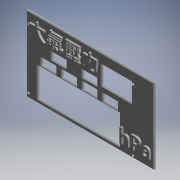
# Autodesk Inventor part: 大氣壓力
Saved by Autodesk Inventor 2021 (Build 250183000, 183)
## iProperties
Part Number: 大氣壓力
Material: 一般
Document SubType Name: 塑型
Designer: aura0
Appearance: 預設
Author: aura0
Autodesk Inventor part; units mm, degrees
ref_plane "YZ 平面" through (0, 0, 0) normal (1, 0, 0) x (0, 1, 0)
ref_plane "XZ 平面" through (0, 0, 0) normal (0, 1, 0) x (-1, 0, 0)
ref_plane "XY 平面" through (0, 0, 0) normal (0, 0, 1) x (1, 0, 0)
sketch "草圖1" plane through (0, 0, 0) normal (0, 0, 1) x (1, 0, 0)
  line L0 (-95, 56.05) -> (95, 56.05)
  line L1 (95, 56.05) -> (95, -56.05)
  line L2 (95, -56.05) -> (-95, -56.05)
  line L3 (-95, -56.05) -> (-95, 56.05)
  line L4 (-95, 56.05) -> (95, -56.05) construction
  line L5 (95, 56.05) -> (-95, -56.05) construction
  point P0 (0, 0)
  dimension "d0" = 190
  dimension "d1" = 112.1
  constraints: 12 end point, 2 midpoint, 2 parallel, 1 horizontal, 1 perpendicular
  measures "d0" distance of L1.end L2.end
  measures "d1" distance of L0.end L1.end
extrude "擠出1" add sketch "草圖1" along normal blind 3
sketch "草圖2" plane through (0, 0, 3) normal (0, 0, 1) x (1, 0, 0)
  line L0 (-78.4, -50.75) -> (43.6, -50.75)
  line L1 (43.6, -50.75) -> (43.6, -7.75)
  line L2 (43.6, -7.75) -> (-78.4, -7.75)
  line L3 (-78.4, -7.75) -> (-78.4, -50.75)
  line L4 (-95, 56.05) -> (-95, -56.05) projected
  line L5 (-95, -56.05) -> (95, -56.05) projected
  line L6 (17.1, 13.68) -> (61.5, 13.68)
  line L7 (61.5, 13.68) -> (61.5, 41.38)
  line L8 (61.5, 41.38) -> (17.1, 41.38)
  line L9 (17.1, 41.38) -> (17.1, 13.68)
  line L10 (-72.8, -5.05) -> (-51.2, -5.05)
  line L11 (-51.2, -5.05) -> (-51.2, 5.15)
  line L12 (-51.2, 5.15) -> (-72.8, 5.15)
  line L13 (-72.8, 5.15) -> (-72.8, -5.05)
  line L14 (-42.2, -5.05) -> (-20.6, -5.05)
  line L15 (-20.6, -5.05) -> (-20.6, 5.15)
  line L16 (-20.6, 5.15) -> (-42.2, 5.15)
  line L17 (-42.2, 5.15) -> (-42.2, -5.05)
  line L18 (-11.6, -5.05) -> (10, -5.05)
  line L19 (10, -5.05) -> (10, 5.15)
  line L20 (10, 5.15) -> (-11.6, 5.15)
  line L21 (-11.6, 5.15) -> (-11.6, -5.05)
  line L22 (19, -5.05) -> (40.6, -5.05)
  line L23 (40.6, -5.05) -> (40.6, 5.15)
  line L24 (40.6, 5.15) -> (19, 5.15)
  line L25 (19, 5.15) -> (19, -5.05)
  line L26 (-57.5, 20.25) -> (-35.9, 20.25)
  line L27 (-35.9, 20.25) -> (-35.9, 10.05)
  line L28 (-35.9, 10.05) -> (-57.5, 10.05)
  line L29 (-57.5, 10.05) -> (-57.5, 20.25)
  line L30 (-11.8, 20.25) -> (9.8, 20.25)
  line L31 (9.8, 20.25) -> (9.8, 10.05)
  line L32 (9.8, 10.05) -> (-11.8, 10.05)
  line L33 (-11.8, 10.05) -> (-11.8, 20.25)
  point P0 (0, 0)
  dimension "d54" = 159
  dimension "d4" = 16.6
  dimension "d5" = 5.3
  dimension "d6" = 122
  dimension "d7" = 43
  dimension "d8" = 51
  dimension "d9" = 22.2
  dimension "d10" = 21.6
  dimension "d11" = 10.2
  dimension "d12" = 21.6
  dimension "d13" = 21.6
  dimension "d14" = 21.6
  dimension "d17" = 10.2
  dimension "d18" = 10.2
  dimension "d19" = 10.2
  dimension "d22" = 9
  dimension "d23" = 9
  dimension "d25" = 9
  dimension "d29" = 37.5
  dimension "d30" = 66.1
  dimension "d31" = 24.1
  dimension "d32" = 10.2
  dimension "d33" = 10.2
  dimension "d34" = 21.6
  dimension "d35" = 21.6
  dimension "d36" = 4.9
  dimension "d37" = 4.9
  dimension "d38" = 69.73
  dimension "d39" = 112.1
  dimension "d40" = 44.4
  dimension "d41" = 27.7
  constraints: 64 end point, 16 parallel, 8 horizontal, 8 perpendicular, 5 point on line
  measures "d4" distance between parallel lines of L4 L3
  measures "d5" distance between parallel lines of L5 L0
  measures "d6" distance of L0.start L0.end
  measures "d7" distance of L2.end L0.start
  measures "d8" distance between parallel lines of L5 L10
  measures "d9" distance between parallel lines of L4 L13
  measures "d10" distance of L10.start L10.end
  measures "d11" distance of L12.end L10.start
  measures "d12" distance of L14.start L14.end
  measures "d13" distance of L18.start L18.end
  measures "d14" distance of L22.start L22.end
  measures "d17" distance of L14.end L15.end
  measures "d18" distance of L18.end L19.end
  measures "d19" distance of L22.end L23.end
  measures "d22" distance between parallel lines of L17 L11
  measures "d23" distance between parallel lines of L21 L15
  measures "d25" distance between parallel lines of L25 L19
  measures "d29" distance between parallel lines of L4 L29
  measures "d30" distance between parallel lines of L5 L28
  measures "d31" distance between parallel lines of L27 L33
  measures "d32" distance of L28.end L26.start
  measures "d33" distance of L32.end L30.start
  measures "d34" distance of L27.end L28.end
  measures "d35" distance of L31.end L32.end
  measures "d36" distance between parallel lines of L16 L28
  measures "d37" distance between parallel lines of L20 L32
  measures "d38" distance between parallel lines of L5 L6
  measures "d39" distance between parallel lines of L4 L9
  measures "d40" distance of L6.start L6.end
  measures "d41" distance of L6.end L7.end
extrude "擠出2" cut sketch "草圖2" against normal blind 3
sketch "草圖3" plane through (0, 0, 3) normal (0, 0, 1) x (1, 0, 0)
  line L0 (-90.6336, 50.0448) -> (-11.3203, 50.0448) construction
  line L1 (-11.3203, 50.0448) -> (-11.3203, 32.4568) construction
  line L2 (-11.3203, 32.4568) -> (-90.6336, 32.4568) construction
  line L3 (-90.6336, 32.4568) -> (-90.6336, 50.0448) construction
  line L4 (44.7132, -22.7639) -> (92.593, -22.7639) construction
  line L5 (92.593, -22.7639) -> (92.593, -44.2402) construction
  line L6 (92.593, -44.2402) -> (44.7132, -44.2402) construction
  line L7 (44.7132, -44.2402) -> (44.7132, -22.7639) construction
  line L8 (-65.6723, 28.4482) -> (-67.0972, 26.5426)
  spline S0 degree 2 poles (-67.0972, 26.5426) (-74.9427, 31.5383) (-77.2774, 39.8302) knots 0 0 0 1 1 1
  spline S1 degree 2 poles (-77.2774, 39.8302) (-79.7495, 31.8474) (-87.595, 26.7315) knots 0 0 0 1 1 1
  line L9 (-87.595, 26.7315) -> (-88.9856, 28.7744)
  spline S2 degree 2 poles (-88.9856, 28.7744) (-80.8997, 34.062) (-79.1315, 41.7186) knots 0 0 0 1 1 1
  line L10 (-79.1315, 41.7186) -> (-88.4362, 41.7186)
  line L11 (-88.4362, 41.7186) -> (-88.4706, 44.0877)
  line L12 (-88.4706, 44.0877) -> (-78.8225, 44.0877)
  spline S3 degree 2 poles (-78.8225, 44.0877) (-78.5306, 46.8688) (-78.4963, 49.7529) knots 0 0 0 1 1 1
  line L13 (-78.4963, 49.7529) -> (-76.1272, 49.7529)
  spline S4 degree 2 poles (-76.1272, 49.7529) (-76.1615, 46.3023) (-76.3504, 44.0877) knots 0 0 0 1 1 1
  line L14 (-76.3504, 44.0877) -> (-66.0156, 44.0877)
  line L15 (-66.0156, 44.0877) -> (-66.0156, 41.7186)
  line L16 (-66.0156, 41.7186) -> (-75.595, 41.7186)
  spline S5 degree 2 poles (-75.595, 41.7186) (-73.6551, 33.2036) (-65.6723, 28.4482) knots 0 0 0 1 1 1
  spline S6 degree 2 poles (-39.0972, 31.9332) (-39.4233, 29.4783) (-40.7967, 26.6456) (-42.05, 26.6456) knots 0 0 0 1 2 2 2
  spline S7 degree 2 poles (-42.05, 26.6456) (-42.8912, 26.6456) (-44.1615, 27.9847) (-45.1229, 33.3238) (-45.1229, 37.3066) knots 0 0 0 1 2 3 3 3
  spline S8 degree 2 poles (-45.1229, 37.3066) (-45.1229, 38.6113) (-45.0542, 39.8817) knots 0 0 0 1 1 1
  line L17 (-45.0542, 39.8817) -> (-59.9555, 39.8817)
  line L18 (-59.9555, 39.8817) -> (-59.9555, 41.8731)
  line L19 (-59.9555, 41.8731) -> (-42.668, 41.8731)
  spline S9 degree 2 poles (-42.668, 41.8731) (-42.7538, 39.6585) (-42.7538, 37.6671) knots 0 0 0 1 1 1
  spline S10 degree 2 poles (-42.7538, 37.6671) (-42.7538, 33.1006) (-42.1015, 29.4268) (-41.8954, 29.4268) knots 0 0 0 1 2 2 2
  spline S11 degree 2 poles (-41.8954, 29.4268) (-41.8096, 29.4268) (-41.2946, 31.3323) (-41.1401, 33.1692) knots 0 0 0 1 2 2 2
  line L20 (-41.1401, 33.1692) -> (-39.0972, 31.9332)
  line L21 (-45.8783, 33.2723) -> (-52.7452, 33.2723)
  line L22 (-52.7452, 33.2723) -> (-52.7452, 26.7486)
  line L23 (-52.7452, 26.7486) -> (-55.0457, 26.7486)
  line L24 (-55.0457, 26.7486) -> (-55.0457, 33.2723)
  line L25 (-55.0457, 33.2723) -> (-61.9469, 33.2723)
  line L26 (-61.9469, 33.2723) -> (-61.9469, 35.2808)
  line L27 (-61.9469, 35.2808) -> (-55.0457, 35.2808)
  line L28 (-55.0457, 35.2808) -> (-55.0457, 39.0233)
  line L29 (-55.0457, 39.0233) -> (-52.7452, 39.0233)
  line L30 (-52.7452, 39.0233) -> (-52.7452, 35.2808)
  line L31 (-52.7452, 35.2808) -> (-45.8783, 35.2808)
  line L32 (-45.8783, 35.2808) -> (-45.8783, 33.2723)
  line L33 (-39.9727, 46.3195) -> (-56.8997, 46.3195)
  spline S12 degree 2 poles (-56.8997, 46.3195) (-58.8568, 43.298) (-60.9341, 41.6843) knots 0 0 0 1 1 1
  line L34 (-60.9341, 41.6843) -> (-62.6165, 43.2808)
  spline S13 degree 2 poles (-62.6165, 43.2808) (-59.698, 45.5984) (-57.4834, 50.0448) knots 0 0 0 1 1 1
  line L35 (-57.4834, 50.0448) -> (-55.1658, 49.4268)
  spline S14 degree 2 poles (-55.1658, 49.4268) (-55.3203, 49.0662) (-55.7324, 48.2765) knots 0 0 0 1 1 1
  line L36 (-55.7324, 48.2765) -> (-39.9727, 48.2765)
  line L37 (-39.9727, 48.2765) -> (-39.9727, 46.3195)
  line L38 (-41.4663, 43.2465) -> (-56.9341, 43.2465)
  line L39 (-56.9341, 43.2465) -> (-56.9341, 45.0147)
  line L40 (-56.9341, 45.0147) -> (-41.4663, 45.0147)
  line L41 (-41.4663, 45.0147) -> (-41.4663, 43.2465)
  spline S15 degree 2 poles (-55.7839, 31.2637) (-57.6723, 29.0147) (-61.0027, 27.1092) knots 0 0 0 1 1 1
  line L42 (-61.0027, 27.1092) -> (-62.6165, 28.8602)
  spline S16 degree 2 poles (-62.6165, 28.8602) (-59.4405, 30.5083) (-57.6379, 32.5856) knots 0 0 0 1 1 1
  line L43 (-57.6379, 32.5856) -> (-55.7839, 31.2637)
  line L44 (-45.6551, 28.7229) -> (-47.3718, 27.2637)
  spline S17 degree 2 poles (-47.3718, 27.2637) (-49.5006, 29.4439) (-51.7667, 31.1435) knots 0 0 0 1 1 1
  line L45 (-51.7667, 31.1435) -> (-50.0156, 32.6371)
  spline S18 degree 2 poles (-50.0156, 32.6371) (-47.6637, 30.9032) (-45.6551, 28.7229) knots 0 0 0 1 1 1
  line L46 (-56.1615, 36.7229) -> (-58.1358, 35.6414)
  spline S19 degree 2 poles (-58.1358, 35.6414) (-59.4405, 37.1006) (-60.7281, 38.1478) knots 0 0 0 1 1 1
  line L47 (-60.7281, 38.1478) -> (-58.7195, 39.298)
  spline S20 degree 2 poles (-58.7195, 39.298) (-57.1057, 38.0105) (-56.1615, 36.7229) knots 0 0 0 1 1 1
  spline S21 degree 2 poles (-47.0113, 38.1135) (-48.1444, 36.7401) (-49.6551, 35.607) knots 0 0 0 1 1 1
  line L48 (-49.6551, 35.607) -> (-51.6122, 36.8259)
  spline S22 degree 2 poles (-51.6122, 36.8259) (-49.9641, 38.1993) (-49.1057, 39.1778) knots 0 0 0 1 1 1
  line L49 (-49.1057, 39.1778) -> (-47.0113, 38.1135)
  line L50 (-12.9341, 47.7959) -> (-32.2645, 47.7959)
  line L51 (-32.2645, 47.7959) -> (-32.2645, 36.2422)
  spline S23 degree 2 poles (-32.2645, 36.2422) (-32.2645, 30.4568) (-34.0843, 26.6113) knots 0 0 0 1 1 1
  line L52 (-34.0843, 26.6113) -> (-35.9555, 28.1564)
  spline S24 degree 2 poles (-35.9555, 28.1564) (-34.4963, 31.7959) (-34.4963, 36.9804) knots 0 0 0 1 1 1
  line L53 (-34.4963, 36.9804) -> (-34.4963, 49.5469)
  line L54 (-34.4963, 49.5469) -> (-12.9341, 49.5469)
  line L55 (-12.9341, 49.5469) -> (-12.9341, 47.7959)
  line L56 (-12.8997, 27.3323) -> (-32.0757, 27.3323)
  line L57 (-32.0757, 27.3323) -> (-32.0757, 29.2379)
  line L58 (-32.0757, 29.2379) -> (-23.6122, 29.2379)
  line L59 (-23.6122, 29.2379) -> (-23.6122, 30.6113)
  line L60 (-23.6122, 30.6113) -> (-30.8912, 30.6113)
  line L61 (-30.8912, 30.6113) -> (-30.8912, 32.4311)
  line L62 (-30.8912, 32.4311) -> (-23.6122, 32.4311)
  line L63 (-23.6122, 32.4311) -> (-23.6122, 33.4954)
  line L64 (-23.6122, 33.4954) -> (-21.2088, 33.4954)
  line L65 (-21.2088, 33.4954) -> (-21.2088, 32.4311)
  line L66 (-21.2088, 32.4311) -> (-14.153, 32.4311)
  line L67 (-14.153, 32.4311) -> (-14.153, 30.6113)
  line L68 (-14.153, 30.6113) -> (-21.2088, 30.6113)
  line L69 (-21.2088, 30.6113) -> (-21.2088, 29.2379)
  line L70 (-21.2088, 29.2379) -> (-12.8997, 29.2379)
  line L71 (-12.8997, 29.2379) -> (-12.8997, 27.3323)
  line L72 (-12.7281, 35.2293) -> (-14.153, 33.6156)
  spline S25 degree 2 poles (-14.153, 33.6156) (-16.0757, 35.4182) (-17.2774, 38.4911) knots 0 0 0 1 1 1
  spline S26 degree 2 poles (-17.2774, 38.4911) (-18.5306, 35.3838) (-20.7281, 33.7014) knots 0 0 0 1 1 1
  line L73 (-20.7281, 33.7014) -> (-21.8439, 35.4868)
  spline S27 degree 2 poles (-21.8439, 35.4868) (-18.9427, 38.1306) (-18.6165, 41.5469) knots 0 0 0 1 1 1
  line L74 (-18.6165, 41.5469) -> (-21.3118, 41.5469)
  line L75 (-21.3118, 41.5469) -> (-21.3118, 43.504)
  line L76 (-21.3118, 43.504) -> (-18.565, 43.504)
  spline S28 degree 2 poles (-18.565, 43.504) (-18.4791, 45.3238) (-18.5135, 46.9375) knots 0 0 0 1 1 1
  line L77 (-18.5135, 46.9375) -> (-16.3504, 46.9375)
  spline S29 degree 2 poles (-16.3504, 46.9375) (-16.3504, 45.3753) (-16.4534, 43.504) knots 0 0 0 1 1 1
  line L78 (-16.4534, 43.504) -> (-13.1916, 43.504)
  line L79 (-13.1916, 43.504) -> (-13.1916, 41.5469)
  line L80 (-13.1916, 41.5469) -> (-16.1615, 41.5469)
  spline S30 degree 2 poles (-16.1615, 41.5469) (-15.4405, 37.5984) (-12.7281, 35.2293) knots 0 0 0 1 1 1
  spline S31 degree 2 poles (-22.3246, 35.7959) (-22.3246, 34.8345) (-23.4577, 33.7873) (-25.7066, 33.9246) knots 0 0 0 1 2 2 2
  line L81 (-25.7066, 33.9246) -> (-26.2216, 35.3152)
  line L82 (-26.2216, 35.3152) -> (-24.7281, 35.3323)
  spline S32 degree 2 poles (-24.7281, 35.3323) (-24.3847, 35.3323) (-24.3847, 35.6929) knots 0 0 0 1 1 1
  line L83 (-24.3847, 35.6929) -> (-24.3847, 36.1907)
  spline S33 degree 2 poles (-24.3847, 36.1907) (-26.565, 35.6757) (-28.4191, 35.4182) knots 0 0 0 1 1 1
  line L84 (-28.4191, 35.4182) -> (-28.7452, 36.2594)
  spline S34 degree 2 poles (-28.7452, 36.2594) (-29.2259, 34.9032) (-30.4963, 33.7529) knots 0 0 0 1 1 1
  line L85 (-30.4963, 33.7529) -> (-32.0585, 35.1263)
  spline S35 degree 2 poles (-32.0585, 35.1263) (-30.5478, 36.4139) (-30.5478, 38.6113) knots 0 0 0 1 1 1
  line L86 (-30.5478, 38.6113) -> (-30.5478, 40.8946)
  line L87 (-30.5478, 40.8946) -> (-22.3246, 40.8946)
  line L88 (-22.3246, 40.8946) -> (-22.3246, 35.7959)
  line L89 (-22.0843, 41.6843) -> (-30.9083, 41.6843)
  line L90 (-30.9083, 41.6843) -> (-30.9083, 46.9375)
  line L91 (-30.9083, 46.9375) -> (-22.0843, 46.9375)
  line L92 (-22.0843, 46.9375) -> (-22.0843, 41.6843)
  line L93 (-24.3847, 37.4611) -> (-24.3847, 39.5727)
  line L94 (-24.3847, 39.5727) -> (-28.4191, 39.5727)
  line L95 (-28.4191, 39.5727) -> (-28.4191, 38.989)
  spline S36 degree 2 poles (-28.4191, 38.989) (-26.3418, 38.9375) (-25.0714, 38.7486) knots 0 0 0 1 1 1
  line L96 (-25.0714, 38.7486) -> (-25.3976, 37.5298)
  spline S37 degree 2 poles (-25.3976, 37.5298) (-26.8568, 37.6843) (-28.4191, 37.7701) knots 0 0 0 1 1 1
  spline S38 degree 2 poles (-28.4191, 37.7701) (-28.4706, 37.1006) (-28.6079, 36.6714) knots 0 0 0 1 1 1
  spline S39 degree 2 poles (-28.6079, 36.6714) (-26.6508, 36.9461) (-24.3847, 37.4611) knots 0 0 0 1 1 1
  line L97 (-13.1401, 44.6027) -> (-14.7882, 43.7787)
  spline S40 degree 2 poles (-14.7882, 43.7787) (-15.2002, 45.0834) (-15.9212, 46.0963) knots 0 0 0 1 1 1
  line L98 (-15.9212, 46.0963) -> (-14.3933, 46.9375)
  spline S41 degree 2 poles (-14.3933, 46.9375) (-13.7581, 46.0791) (-13.1401, 44.6027) knots 0 0 0 1 1 1
  line L99 (-24.213, 43.0062) -> (-24.213, 43.7444)
  line L100 (-24.213, 43.7444) -> (-28.7452, 43.7444)
  line L101 (-28.7452, 43.7444) -> (-28.7452, 43.0062)
  line L102 (-28.7452, 43.0062) -> (-24.213, 43.0062)
  line L103 (-24.213, 44.9461) -> (-24.213, 45.6499)
  line L104 (-24.213, 45.6499) -> (-28.7452, 45.6499)
  line L105 (-28.7452, 45.6499) -> (-28.7452, 44.9461)
  line L106 (-28.7452, 44.9461) -> (-24.213, 44.9461)
  spline S42 degree 2 poles (12.2676, 45.3238) (12.2333, 38.2508) (11.6496, 29.6156) (10.5852, 27.5727) (8.8513, 26.7143) (5.8299, 26.7143) knots 0 0 0 1 2 3 4 4 4
  spline S43 degree 2 poles (5.8299, 26.7143) (4.92, 26.7143) (4.0616, 26.7486) knots 0 0 0 1 1 1
  line L107 (4.0616, 26.7486) -> (3.1689, 29.2036)
  spline S44 degree 2 poles (3.1689, 29.2036) (4.4737, 29.1349) (7.5466, 29.1349) knots 0 0 0 1 1 1
  spline S45 degree 2 poles (7.5466, 29.1349) (8.0616, 29.1349) (8.8513, 29.6671) (9.1603, 30.4911) (9.5895, 35.6242) (9.6754, 38.1821) knots 0 0 0 1 2 3 4 4 4
  line L108 (9.6754, 38.1821) -> (9.8299, 43.0577)
  line L109 (9.8299, 43.0577) -> (2.1561, 43.0577)
  spline S46 degree 2 poles (2.1561, 43.0577) (1.7784, 36.7916) (-2.8053, 29.5469) (-7.8354, 26.6971) knots 0 0 0 1 2 2 2
  line L110 (-7.8354, 26.6971) -> (-9.4148, 28.6542)
  spline S47 degree 2 poles (-9.4148, 28.6542) (-5.7066, 30.4396) (-0.6594, 36.5856) (-0.213, 43.0577) knots 0 0 0 1 2 2 2
  line L111 (-0.213, 43.0577) -> (-8.5907, 43.0577)
  line L112 (-8.5907, 43.0577) -> (-8.5907, 45.3238)
  line L113 (-8.5907, 45.3238) -> (-0.0929, 45.3238)
  spline S48 degree 2 poles (-0.0929, 45.3238) (0.0616, 47.401) (0.0273, 49.8903) knots 0 0 0 1 1 1
  line L114 (0.0273, 49.8903) -> (2.4479, 49.8903)
  spline S49 degree 2 poles (2.4479, 49.8903) (2.4479, 47.9332) (2.2934, 45.3238) knots 0 0 0 1 1 1
  line L115 (2.2934, 45.3238) -> (12.2676, 45.3238)
  line L116 (59.3569, -43.8969) -> (56.3355, -43.8969)
  line L117 (56.3355, -43.8969) -> (56.3355, -35.7081)
  spline S50 degree 2 poles (56.3355, -35.7081) (56.3355, -31.7081) (53.3827, -31.7081) knots 0 0 0 1 1 1
  spline S51 degree 2 poles (53.3827, -31.7081) (51.872, -31.7081) (49.8977, -34.0085) (49.8977, -35.7939) knots 0 0 0 1 2 2 2
  line L118 (49.8977, -35.7939) -> (49.8977, -43.8969)
  line L119 (49.8977, -43.8969) -> (46.8591, -43.8969)
  line L120 (46.8591, -43.8969) -> (46.8591, -22.7639)
  line L121 (46.8591, -22.7639) -> (49.8977, -22.7639)
  line L122 (49.8977, -22.7639) -> (49.8977, -31.8969)
  line L123 (49.8977, -31.8969) -> (49.9492, -31.8969)
  spline S52 degree 2 poles (49.9492, -31.8969) (51.5801, -29.2875) (54.5329, -29.2875) knots 0 0 0 1 1 1
  spline S53 degree 2 poles (54.5329, -29.2875) (59.3569, -29.2875) (59.3569, -35.1244) knots 0 0 0 1 1 1
  line L124 (59.3569, -35.1244) -> (59.3569, -43.8969)
  line L125 (66.8419, -36.5836) -> (66.8419, -43.8969)
  line L126 (66.8419, -43.8969) -> (63.7518, -43.8969)
  line L127 (63.7518, -43.8969) -> (63.7518, -23.8969)
  line L128 (63.7518, -23.8969) -> (69.7947, -23.8969)
  spline S54 degree 2 poles (69.7947, -23.8969) (73.1938, -23.8969) (76.799, -27.0385) (76.799, -30.0257) knots 0 0 0 1 2 2 2
  spline S55 degree 2 poles (76.799, -30.0257) (76.799, -33.0299) (72.49, -36.6866) (69.314, -36.5836) knots 0 0 0 1 2 2 2
  line L129 (69.314, -36.5836) -> (66.8419, -36.5836)
  line L130 (66.8419, -26.4892) -> (66.8419, -33.9913)
  line L131 (66.8419, -33.9913) -> (69.0737, -33.9913)
  spline S56 degree 2 poles (69.0737, -33.9913) (73.5544, -33.9913) (73.5544, -30.1458) knots 0 0 0 1 1 1
  spline S57 degree 2 poles (73.5544, -30.1458) (73.5544, -26.4892) (69.2453, -26.4892) knots 0 0 0 1 1 1
  line L132 (69.2453, -26.4892) -> (66.8419, -26.4892)
  spline S58 degree 2 poles (80.2668, -30.575) (82.4471, -29.2875) (85.314, -29.2875) knots 0 0 0 1 1 1
  spline S59 degree 2 poles (85.314, -29.2875) (90.7217, -29.2875) (90.7217, -34.8669) knots 0 0 0 1 1 1
  line L133 (90.7217, -34.8669) -> (90.7217, -43.8969)
  line L134 (90.7217, -43.8969) -> (87.7861, -43.8969)
  line L135 (87.7861, -43.8969) -> (87.7861, -41.7338)
  line L136 (87.7861, -41.7338) -> (87.7174, -41.7338)
  spline S60 degree 2 poles (87.7174, -41.7338) (86.2582, -44.2402) (83.3741, -44.2402) knots 0 0 0 1 1 1
  spline S61 degree 2 poles (83.3741, -44.2402) (81.2797, -44.2402) (78.8591, -41.957) (78.8591, -40.0342) knots 0 0 0 1 2 2 2
  spline S62 degree 2 poles (78.8591, -40.0342) (78.8591, -36.0171) (83.6488, -35.3304) knots 0 0 0 1 1 1
  line L137 (83.6488, -35.3304) -> (87.8033, -34.7639)
  spline S63 degree 2 poles (87.8033, -34.7639) (87.8033, -31.5879) (84.9878, -31.5879) knots 0 0 0 1 1 1
  spline S64 degree 2 poles (84.9878, -31.5879) (82.4299, -31.5879) (80.2668, -33.2531) knots 0 0 0 1 1 1
  line L138 (80.2668, -33.2531) -> (80.2668, -30.575)
  spline S65 degree 2 poles (84.6445, -37.2531) (83.0994, -37.4763) (81.8119, -38.6265) (81.8119, -39.7596) knots 0 0 0 1 2 2 2
  spline S66 degree 2 poles (81.8119, -39.7596) (81.8119, -40.7038) (83.1853, -41.8883) (84.2496, -41.8883) knots 0 0 0 1 2 2 2
  spline S67 degree 2 poles (84.2496, -41.8883) (85.7775, -41.8883) (87.8033, -39.7424) (87.8033, -38.0943) knots 0 0 0 1 2 2 2
  line L139 (87.8033, -38.0943) -> (87.8033, -36.8411)
  line L140 (87.8033, -36.8411) -> (84.6445, -37.2531)
  point P0 (0, 0)
  constraints: 4 other
extrude "擠出3" add sketch "草圖3" along normal blind 3
sketch "草圖4" plane through (0, 0, 3) normal (0, 0, 1) x (1, 0, 0)
  circle A0 centre (-91.6, 39.45) radius 1.8
  circle A1 centre (-91.6, -49.55) radius 1.8
  circle A2 centre (64, 39.45) radius 1.8
  circle A3 centre (64, -52.65) radius 1.8
  line L0 (-95, 56.05) -> (-95, -56.05) projected
  line L1 (-95, -56.05) -> (95, -56.05) projected
  point P0 (0, 0)
  dimension "d46" = 3.4
  dimension "d47" = 6.5
  dimension "d48" = 3.6
  dimension "d49" = 95.5
  dimension "d50" = 3.4
  dimension "d51" = 3.6
  dimension "d52" = 3.6
  dimension "d53" = 3.6
  dimension "d54" = 159
  dimension "d55" = 3.4
  dimension "d56" = 95.5
  dimension "d57" = 159
  constraints: 4 centre point
  measures "d46" distance from line of L0 A1.centre
  measures "d47" distance from line of L1 A1.centre
  measures "d48" diameter of A1
  measures "d49" distance from line of L1 A0.centre
  measures "d50" distance from line of L0 A0.centre
  measures "d51" diameter of A0
  measures "d52" diameter of A2
  measures "d53" diameter of A3
  measures "d54" distance from line of L0 A3.centre
  measures "d55" distance from line of L1 A3.centre
  measures "d56" distance from line of L1 A2.centre
  measures "d57" distance from line of L0 A2.centre
extrude "擠出4" cut sketch "草圖4" against normal blind 3
chamfer "倒角1" distance 1 angle 45 36 edges at (0, 56.05, 3) (-95, 0, 3) (0, -56.05, 3) (-17.4, -50.75, 3) (-78.4, -29.25, 3) (-17.4, -7.75, 3) (43.6, -29.25, 3) (29.8, -5.05, 3) (19, 0.05, 3) (29.8, 5.15, 3) (40.6, 0.05, 3) (10, 0.05, 3) (-0.8, 5.15, 3) (-11.6, 0.05, 3) (-0.8, -5.05, 3) (-20.6, 0.05, 3) (-31.4, 5.15, 3) (-42.2, 0.05, 3) (-31.4, -5.05, 3) (-51.2, 0.05, 3) (-62, 5.15, 3) (-72.8, 0.05, 3) (-62, -5.05, 3) (-57.5, 15.15, 3) (-46.7, 20.25, 3) (-35.9, 15.15, 3) (-46.7, 10.05, 3) (-11.8, 15.15, 3) (-1, 20.25, 3) (9.8, 15.15, 3) (-1, 10.05, 3) (17.1, 27.53, 3) (39.3, 13.68, 3) (39.3, 41.38, 3) (95, 0, 3) (61.5, 27.53, 3)
equation "\"d12\" = d10"
equation "\"d13\" = d12"
equation "\"d14\" = d13"
equation "\"d17\" = d11"
equation "\"d32\" = d11"
equation "\"d33\" = d11"
equation "\"d34\" = d10"
equation "\"d35\" = d10"
equation "\"d37\" = d36"
equation "\"d50\" = d46"
equation "\"d51\" = d48"
equation "\"d52\" = d48"
equation "\"d53\" = d48"
equation "\"d55\" = d46"
equation "\"d56\" = d49"
equation "\"d57\" = d54"
